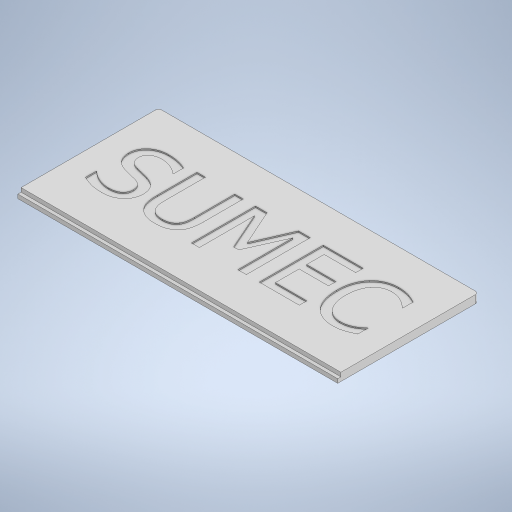
# Autodesk Inventor part: Kryt těla
Saved by Autodesk Inventor 2023.2 (Build 272271030, 271C)
## iProperties
Created: 2023-03-18
Part Number: Kryt těla
Material: Všeobecné
Document SubType Name: Modeling
Designer: jaryj
Density: 1 g/cm^3
Appearance: Výchozí
Author: jaryj
Autodesk Inventor part; units mm, degrees
ref_plane "YZ Plane" through (0, 0, 0) normal (1, 0, 0) x (0, 1, 0)
ref_plane "XZ Plane" through (0, 0, 0) normal (0, 1, 0) x (-1, 0, 0)
ref_plane "XY Plane" through (0, 0, 0) normal (0, 0, 1) x (1, 0, 0)
sketch "Náčrt1" plane through (0, 0, 0) normal (0, 1, 0) x (-1, 0, 0)
  line L0 (0, 0) -> (50, 0)
  line L1 (50, 0) -> (50, -44)
  line L2 (50, -44) -> (0, -44)
  line L3 (0, -44) -> (0, 0)
  line L4 (0, -1) -> (50, -1)
  line L5 (18, -41) -> (16, -41)
  line L6 (18, -41) -> (18, -43.9)
  line L7 (18, -43.9) -> (16, -43.9)
  line L8 (16, -43.9) -> (16, -41)
  line L9 (5.25, -44) -> (5.25, -40)
  line L10 (5.25, -40) -> (9.75, -40)
  line L11 (9.75, -40) -> (9.75, -44)
  dimension "d0" = 44
  dimension "d1" = 50
  dimension "d2" = 1
  dimension "d5" = 3
  dimension "d16" = 0.1
  dimension "d17" = 32
  dimension "d18" = 2
  dimension "d28" = 4.5
  dimension "d29" = 4
  dimension "d30" = 5.25
  constraints: 24 end point, 7 perpendicular, 4 point on line, 2 parallel, 1 horizontal, 1 vertical
  measures "d0" distance of L2.end L0.start
  measures "d1" distance of L1.end L2.end
  measures "d2" distance between parallel lines of L0 L4
  measures "d5" distance between parallel lines of L2 L5
  measures "d16" distance between parallel lines of L2 L7
  measures "d17" distance from line of L1 L5.start
  measures "d18" distance of L5.start L5.end
  measures "d28" distance of L9.end L10.end
  measures "d29" distance of L10.end L11.end
  measures "d30" distance between parallel lines of L3 L9
extrude "Vysunutí1" add sketch "Náčrt1" along normal blind 2.5 contours L4 L1 L2 L11 L10 L9 L3 | L9 L10 L11 L2 | L6 L7 L8 L5
extrude "Vysunutí2" add sketch "Náčrt1" along normal blind 1.25 contours L0 L1 L4 L3
extrude "Vysunutí3" add sketch "Náčrt1" against normal blind 7.5 contours L6 L7 L8 L5
sketch "Náčrt3" plane through (-16, 0, -43.9) normal (0, 0, -1) x (-1, 0, 0)
  line L0 (0, 0) -> (0, -7.5) projected
  line L1 (2, -7.5) -> (0, -7.5) projected
  line L2 (2, 0) -> (2, -7.5) projected
  line L3 (0, 0) -> (0, -7.5) projected
  line L4 (0, -5.6) -> (2, -5.6)
  line L5 (2, 0) -> (2, -7.5) projected
  point P0 (-16, 0)
  dimension "d19" = 1.9
  constraints: 2 end point, 2 point on line, 1 perpendicular
  measures "d19" distance between parallel lines of L4 L1
extrude "Vysunutí5" add sketch "Náčrt3" along normal blind 5
fillet "Zaoblení1" radius 1 1 edges at (-50, 1.25, -44)
extrude "Vysunutí6" add sketch "Náčrt1" against normal blind 8 contours L9 L10 L11 L2
sketch "Náčrt7" plane through (-5.25, -8, -40) normal (1, 0, 0) x (0, 0, -1)
  line L0 (0, 8) -> (0, 0) projected
  line L1 (4, 0) -> (0, 0) projected
  line L2 (4, 8) -> (4, 0) projected
  line L3 (0, 8) -> (0, 0) projected
  line L4 (0, 2) -> (4, 2)
  line L5 (4, 8) -> (4, 0) projected
  point P0 (-40, 8)
  dimension "d36" = 2
  constraints: 2 end point, 2 point on line, 1 perpendicular
  measures "d36" distance between parallel lines of L1 L4
extrude "Vysunutí8" add sketch "Náčrt7" along normal up to surface (5.25 mm away)
sketch "Náčrt8" plane through (0, 0, -44) normal (0, 0, -1) x (-1, 0, 0)
  line L0 (9.75, 0) -> (9.75, -8) projected
  line L1 (5.25, -6) -> (0, -6) projected
  point P0 (0, 0)
  point P1 (7.5, -3)
  dimension "d46" = 2.25
  dimension "d47" = 3
  measures "d46" distance from line of L0 point (7.5, -3)
  measures "d47" distance from line of L1 point (7.5, -3)
hole "Díra1" at (-7.5, -3, -44) direction (0, 0, 1) diameter 2 end through all
mirror "Zrcadlit2" about plane through (0, 0, -1) normal (1, 0, 0)
sketch "Náčrt4" plane through (0, 2.5, 0) normal (0, 1, 0) x (1, 0, 0)
  line L0 (-43.75, 33) -> (41.25, 33) construction
  line L1 (41.25, 33) -> (41.25, 13) construction
  line L2 (41.25, 13) -> (-43.75, 13) construction
  line L3 (-43.75, 13) -> (-43.75, 33) construction
  line L4 (-49, 44) -> (49, 44) projected
  line L5 (-50, 43) -> (-50, 1) projected
  spline S0 degree 2 poles (-36.1487, 12.2869) (-38.3205, 12.2869) (-41.3675, 13.1945) (-42.7127, 13.8428) knots 0 0 0 1 2 2 2
  line L6 (-42.7127, 13.8428) -> (-42.7127, 17.1815)
  line L7 (-42.7127, 17.1815) -> (-42.5182, 17.1815)
  spline S1 degree 2 poles (-42.5182, 17.1815) (-41.2054, 15.9498) (-37.8829, 14.5883) (-36.3432, 14.5883) knots 0 0 0 1 2 2 2
  spline S2 degree 2 poles (-36.3432, 14.5883) (-34.139, 14.5883) (-31.8861, 16.4198) (-31.8861, 17.9271) knots 0 0 0 1 2 2 2
  spline S3 degree 2 poles (-31.8861, 17.9271) (-31.8861, 19.1264) (-33.0693, 20.6175) (-34.3497, 20.9903) knots 0 0 0 1 2 2 2
  spline S4 degree 2 poles (-34.3497, 20.9903) (-35.2735, 21.2496) (-36.8132, 21.6062) (-37.9639, 21.8979) knots 0 0 0 1 2 2 2
  spline S5 degree 2 poles (-37.9639, 21.8979) (-39.0012, 22.1734) (-40.6382, 23) (-41.2703, 23.6645) knots 0 0 0 1 2 2 2
  spline S6 degree 2 poles (-41.2703, 23.6645) (-41.8861, 24.329) (-42.5669, 26.1118) (-42.5669, 27.2788) knots 0 0 0 1 2 2 2
  spline S7 degree 2 poles (-42.5669, 27.2788) (-42.5669, 29.7099) (-38.7743, 33) (-35.8408, 33) knots 0 0 0 1 2 2 2
  spline S8 degree 2 poles (-35.8408, 33) (-34.1552, 33) (-31.173, 32.3355) (-29.8926, 31.7034) knots 0 0 0 1 2 2 2
  line L8 (-29.8926, 31.7034) -> (-29.8926, 28.5267)
  line L9 (-29.8926, 28.5267) -> (-30.0871, 28.5267)
  spline S9 degree 2 poles (-30.0871, 28.5267) (-31.0434, 29.4019) (-34.0255, 30.6985) (-35.6625, 30.6985) knots 0 0 0 1 2 2 2
  spline S10 degree 2 poles (-35.6625, 30.6985) (-37.5101, 30.6985) (-39.7954, 28.9643) (-39.7954, 27.5543) knots 0 0 0 1 2 2 2
  spline S11 degree 2 poles (-39.7954, 27.5543) (-39.7954, 26.2901) (-38.4502, 24.7828) (-37.186, 24.4425) knots 0 0 0 1 2 2 2
  spline S12 degree 2 poles (-37.186, 24.4425) (-36.3432, 24.2156) (-33.8959, 23.6321) (-33.0855, 23.389) knots 0 0 0 1 2 2 2
  spline S13 degree 2 poles (-33.0855, 23.389) (-31.0271, 22.7569) (-29.1147, 20.2123) (-29.1147, 18.3485) knots 0 0 0 1 2 2 2
  spline S14 degree 2 poles (-29.1147, 18.3485) (-29.1147, 17.1653) (-30.0709, 14.8963) (-30.9299, 14.1021) knots 0 0 0 1 2 2 2
  spline S15 degree 2 poles (-30.9299, 14.1021) (-31.8861, 13.2269) (-34.3173, 12.2869) (-36.1487, 12.2869) knots 0 0 0 1 2 2 2
  spline S16 degree 2 poles (-19.4226, 12.222) (-21.1892, 12.222) (-23.8148, 13.1459) (-24.7387, 14.0697) knots 0 0 0 1 2 2 2
  spline S17 degree 2 poles (-24.7387, 14.0697) (-25.7921, 15.107) (-26.6511, 18.0243) (-26.6511, 20.1637) knots 0 0 0 1 2 2 2
  line L10 (-26.6511, 20.1637) -> (-26.6511, 32.6434)
  line L11 (-26.6511, 32.6434) -> (-23.9931, 32.6434)
  line L12 (-23.9931, 32.6434) -> (-23.9931, 20.1637)
  spline S18 degree 2 poles (-23.9931, 20.1637) (-23.9931, 18.7699) (-23.6365, 16.8898) (-23.1341, 16.128) knots 0 0 0 1 2 2 2
  spline S19 degree 2 poles (-23.1341, 16.128) (-22.5993, 15.3177) (-20.7516, 14.4911) (-19.4226, 14.4911) knots 0 0 0 1 2 2 2
  spline S20 degree 2 poles (-19.4226, 14.4911) (-18.1746, 14.4911) (-16.2297, 15.3177) (-15.6949, 16.128) knots 0 0 0 1 2 2 2
  spline S21 degree 2 poles (-15.6949, 16.128) (-15.1925, 16.8898) (-14.8359, 18.7536) (-14.8359, 20.0989) knots 0 0 0 1 2 2 2
  line L13 (-14.8359, 20.0989) -> (-14.8359, 32.6434)
  line L14 (-14.8359, 32.6434) -> (-12.1779, 32.6434)
  line L15 (-12.1779, 32.6434) -> (-12.1779, 20.1637)
  spline S22 degree 2 poles (-12.1779, 20.1637) (-12.1779, 18.0729) (-13.0207, 15.0908) (-14.0904, 14.0697) knots 0 0 0 1 2 2 2
  spline S23 degree 2 poles (-14.0904, 14.0697) (-15.0466, 13.1297) (-17.575, 12.222) (-19.4226, 12.222) knots 0 0 0 1 2 2 2
  line L16 (8.7784, 12.6434) -> (6.1203, 12.6434)
  line L17 (6.1203, 12.6434) -> (6.1203, 29.872)
  line L18 (6.1203, 29.872) -> (0.9015, 18.154)
  line L19 (0.9015, 18.154) -> (-0.7192, 18.154)
  line L20 (-0.7192, 18.154) -> (-5.8894, 29.872)
  line L21 (-5.8894, 29.872) -> (-5.8894, 12.6434)
  line L22 (-5.8894, 12.6434) -> (-8.3691, 12.6434)
  line L23 (-8.3691, 12.6434) -> (-8.3691, 32.6434)
  line L24 (-8.3691, 32.6434) -> (-4.7387, 32.6434)
  line L25 (-4.7387, 32.6434) -> (0.2532, 21.5089)
  line L26 (0.2532, 21.5089) -> (5.0831, 32.6434)
  line L27 (5.0831, 32.6434) -> (8.7784, 32.6434)
  line L28 (8.7784, 32.6434) -> (8.7784, 12.6434)
  line L29 (12.8302, 12.6434) -> (12.8302, 32.6434)
  line L30 (12.8302, 32.6434) -> (25.3424, 32.6434)
  line L31 (25.3424, 32.6434) -> (25.3424, 30.2771)
  line L32 (25.3424, 30.2771) -> (15.4882, 30.2771)
  line L33 (15.4882, 30.2771) -> (15.4882, 24.799)
  line L34 (15.4882, 24.799) -> (24.6779, 24.799)
  line L35 (24.6779, 24.799) -> (24.6779, 22.4327)
  line L36 (24.6779, 22.4327) -> (15.4882, 22.4327)
  line L37 (15.4882, 22.4327) -> (15.4882, 15.0097)
  line L38 (15.4882, 15.0097) -> (25.3424, 15.0097)
  line L39 (25.3424, 15.0097) -> (25.3424, 12.6434)
  line L40 (25.3424, 12.6434) -> (12.8302, 12.6434)
  spline S24 degree 2 poles (36.0717, 12.2869) (34.1268, 12.2869) (30.8367, 13.5997) (29.6374, 14.9125) knots 0 0 0 1 2 2 2
  spline S25 degree 2 poles (29.6374, 14.9125) (28.438, 16.2091) (27.1252, 20.0989) (27.1252, 22.6272) knots 0 0 0 1 2 2 2
  spline S26 degree 2 poles (27.1252, 22.6272) (27.1252, 25.1394) (28.4056, 28.8671) (29.6212, 30.2447) knots 0 0 0 1 2 2 2
  spline S27 degree 2 poles (29.6212, 30.2447) (30.8205, 31.59) (34.0944, 33) (36.1203, 33) knots 0 0 0 1 2 2 2
  spline S28 degree 2 poles (36.1203, 33) (37.1252, 33) (38.8918, 32.7083) (39.6374, 32.4814) knots 0 0 0 1 2 2 2
  spline S29 degree 2 poles (39.6374, 32.4814) (40.2857, 32.2707) (41.6309, 31.671) (42.2954, 31.3144) knots 0 0 0 1 2 2 2
  line L41 (42.2954, 31.3144) -> (42.2954, 28.1053)
  line L42 (42.2954, 28.1053) -> (42.0847, 28.1053)
  spline S30 degree 2 poles (42.0847, 28.1053) (41.7281, 28.4295) (40.626, 29.3371) (39.8318, 29.7747) knots 0 0 0 1 2 2 2
  spline S31 degree 2 poles (39.8318, 29.7747) (39.0701, 30.1961) (37.2711, 30.731) (36.1041, 30.731) knots 0 0 0 1 2 2 2
  spline S32 degree 2 poles (36.1041, 30.731) (34.8237, 30.731) (32.5385, 29.6775) (31.6795, 28.6726) knots 0 0 0 1 2 2 2
  spline S33 degree 2 poles (31.6795, 28.6726) (30.8367, 27.6515) (29.8967, 24.5559) (29.8967, 22.6272) knots 0 0 0 1 2 2 2
  spline S34 degree 2 poles (29.8967, 22.6272) (29.8967, 20.5689) (30.8853, 17.6029) (31.7443, 16.5818) knots 0 0 0 1 2 2 2
  spline S35 degree 2 poles (31.7443, 16.5818) (32.5871, 15.5932) (34.84, 14.5883) (36.1041, 14.5883) knots 0 0 0 1 2 2 2
  spline S36 degree 2 poles (36.1041, 14.5883) (37.2549, 14.5883) (39.216, 15.1556) (39.9777, 15.577) knots 0 0 0 1 2 2 2
  spline S37 degree 2 poles (39.9777, 15.577) (40.7071, 15.9984) (41.7929, 16.8736) (42.1009, 17.1815) knots 0 0 0 1 2 2 2
  line L43 (42.1009, 17.1815) -> (42.2954, 17.1815)
  line L44 (42.2954, 17.1815) -> (42.2954, 14.0049)
  spline S38 degree 2 poles (42.2954, 14.0049) (41.6309, 13.6969) (40.4639, 13.1297) (39.6374, 12.8703) knots 0 0 0 1 2 2 2
  spline S39 degree 2 poles (39.6374, 12.8703) (38.7622, 12.5786) (37.2711, 12.2869) (36.0717, 12.2869) knots 0 0 0 1 2 2 2
  point P0 (0, 0)
  dimension "d22" = 85
  dimension "d23" = 20
  dimension "d24" = 11
  dimension "d25" = 6.25
  constraints: 2 other
  measures "d22" distance of L1.end L2.end
  measures "d23" distance of L0.end L1.end
  measures "d24" distance between parallel lines of L4 L0
  measures "d25" distance between parallel lines of L5 L3
emboss "Reliéf1" sketch "Náčrt4" operation cut depth 0.4 direction (0, -1, 0)
